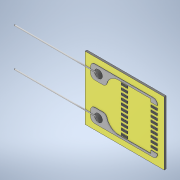
# Autodesk Inventor part: 應變規
Saved by Autodesk Inventor 2022 (Build 260153000, 153)
## iProperties
Created: 2023-03-14
Part Number: 應變規
Material: 一般
Document SubType Name: Modeling
Designer: User
Mass: 0.168829 g
Surface Area: 7.27926 cm^2
Volume: 0.168829 cm^3
Density: 1 g/cm^3
Appearance: 預設
Author: User
Autodesk Inventor part; units mm, degrees
ref_plane "XZ Plane" through (0, 0, 0) normal (0, 1, 0) x (-1, 0, 0)
ref_plane "XY Plane" through (0, 0, 0) normal (0, 0, 1) x (1, 0, 0)
sketch "草圖1" plane through (0, 0, 0) normal (0, 0, 1) x (1, 0, 0)
  line L0 (-10, 8) -> (10, 8)
  line L1 (10, 8) -> (10, -8)
  line L2 (10, -8) -> (-10, -8)
  line L3 (-10, -8) -> (-10, 8)
  line L4 (-14, 0) -> (14, 0) construction
  line L5 (0, -11.2) -> (0, 11.2) construction
  point P0 (0, 0)
  point P1 (0, 8)
  point P2 (10, 0)
  dimension "d0" = 16
  dimension "d1" = 20
  constraints: 8 end point, 2 midpoint, 2 parallel, 2 point on line, 1 horizontal, 1 perpendicular
  measures "d0" distance of L0.end L1.end
  measures "d1" distance of L0.start L0.end
extrude "擠出1" add sketch "草圖1" along normal blind 0.5
sketch "草圖2" plane through (0, 0, 0.5) normal (0, 0, 1) x (1, 0, 0)
  line L0 (-8, 6) -> (8, 6)
  line L1 (8, -6) -> (-8, -6)
  line L2 (-8, 6) -> (-4.5, 6)
  line L3 (-4.5, 6) -> (-4.5, 3)
  line L4 (-4.5, 3) -> (-8, 3)
  line L5 (-8, 3) -> (-8, 6)
  line L6 (-8, -6) -> (-4.5, -6)
  line L7 (-4.5, -6) -> (-4.5, -3)
  line L8 (-4.5, -3) -> (-8, -3)
  line L9 (-8, -3) -> (-8, -6)
  arc A0 (-1.5, 6) -> (-4.5, 3) centre (-1.5, 3) ccw
  arc A1 (-4.5, -3) -> (-1.5, -6) centre (-1.5, -3) ccw
  line L10 (-14, 0) -> (14, 0) construction
  line L11 (0, -11.2) -> (0, 11.2) construction
  line L12 (-8.5, 6.5) -> (8.3, 6.5)
  line L13 (8.3, -6.5) -> (-8.5, -6.5)
  line L14 (-8, 3) -> (-8.5, 3)
  line L15 (-8, -3) -> (-8.5, -3)
  line L16 (-8, -6) -> (-8, -3)
  line L17 (-8, 3) -> (-8, 6)
  line L18 (-8.5, 6.5) -> (-8.5, 3)
  line L19 (-8.5, -3) -> (-8.5, -6.5)
  line L20 (8.3, 6.5) -> (6.7, 6.5)
  line L21 (6.7, 6.5) -> (6.7, 5.5)
  line L22 (6.7, 5.5) -> (8.3, 5.5)
  line L23 (8.3, 5.5) -> (8.3, 6.5)
  line L24 (8.3, -6.5) -> (6.7, -6.5)
  line L25 (6.7, -6.5) -> (6.7, -5.5)
  line L26 (6.7, -5.5) -> (8.3, -5.5)
  line L27 (8.3, -5.5) -> (8.3, -6.5)
  line L28 (8.3, 6.5) -> (8.3, 5.5)
  line L29 (8.3, -5.5) -> (8.3, -6.5)
  line L30 (8.3, 6) -> (8.3, 5.5)
  line L31 (8.3, -5.5) -> (8.3, -6)
  line L32 (8, 6) -> (8, 5.5)
  line L33 (8, -5.5) -> (8, -6)
  line L34 (8, -6) -> (8, -5.5)
  line L35 (8, 5.5) -> (8, 6)
  point P0 (0, 0)
  point P1 (0, 6)
  point P2 (6.7, 6)
  point P3 (6.7, -6)
  dimension "d5" = 12
  dimension "d6" = 3
  dimension "d7" = 3
  dimension "d8" = 3.5
  dimension "d9" = 0.5
  dimension "d41" = 1
  dimension "d42" = 1
  dimension "d43" = 1.6
  dimension "d44" = 1.6
  constraints: 68 end point, 18 parallel, 12 perpendicular, 6 point on line, 5 horizontal, 4 point on circle, 4 tangent, 2 centre point, 2 midpoint, 2 vertical
  measures "d5" distance between parallel lines of L1 L0
  measures "d6" distance between parallel lines of L0 L4
  measures "d7" distance between parallel lines of L6 L8
  measures "d8" distance between parallel lines of L5 L3
  measures "d9" distance between parallel lines of L12 L0
  measures "d41" distance between parallel lines of L20 L22
  measures "d42" distance between parallel lines of L13 L26
  measures "d43" distance of L26.end L25.end
  measures "d44" distance of L21.end L22.end
extrude "擠出2" add sketch "草圖2" along normal blind 0.1
fillet "圓角1" radius 1 6 edges at (-4.5, 3, 0.55) (-4.5, -3, 0.55) (-8.5, -3, 0.55) (-8.5, 3, 0.55) (-8.5, 6.5, 0.55) (-8.5, -6.5, 0.55)
fillet "圓角2" radius 1 2 edges at (8.3, 6.5, 0.55) (8.3, -6.5, 0.55)
sketch "草圖3" plane through (0, 0, 0.5) normal (0, 0, 1) x (1, 0, 0)
  line L0 (0, -11.2) -> (0, 11.2) construction
  line L1 (-14, 0) -> (14, 0) construction
  line L2 (-0.8, 5.75) -> (0.8, 5.75)
  line L3 (0.8, 5.75) -> (0.8, 5.25)
  line L4 (0.8, 5.25) -> (-0.8, 5.25)
  line L5 (-0.8, 5.25) -> (-0.8, 5.75)
  line L6 (-0.8, 4.65) -> (0.8, 4.65)
  line L7 (0.8, 4.65) -> (0.8, 4.15)
  line L8 (0.8, 4.15) -> (-0.8, 4.15)
  line L9 (-0.8, 4.15) -> (-0.8, 4.65)
  line L10 (-0.8, 3.55) -> (0.8, 3.55)
  line L11 (0.8, 3.55) -> (0.8, 3.05)
  line L12 (0.8, 3.05) -> (-0.8, 3.05)
  line L13 (-0.8, 3.05) -> (-0.8, 3.55)
  line L14 (-0.8, 2.45) -> (0.8, 2.45)
  line L15 (0.8, 2.45) -> (0.8, 1.95)
  line L16 (0.8, 1.95) -> (-0.8, 1.95)
  line L17 (-0.8, 1.95) -> (-0.8, 2.45)
  line L18 (-0.8, 1.35) -> (0.8, 1.35)
  line L19 (0.8, 1.35) -> (0.8, 0.85)
  line L20 (0.8, 0.85) -> (-0.8, 0.85)
  line L21 (-0.8, 0.85) -> (-0.8, 1.35)
  line L22 (-0.8, 0.25) -> (0.8, 0.25)
  line L23 (0.8, 0.25) -> (0.8, -0.25)
  line L24 (0.8, -0.25) -> (-0.8, -0.25)
  line L25 (-0.8, -0.25) -> (-0.8, 0.25)
  line L26 (-0.8, -5.75) -> (0.8, -5.75)
  line L27 (0.8, -5.75) -> (0.8, -5.25)
  line L28 (0.8, -5.25) -> (-0.8, -5.25)
  line L29 (-0.8, -5.25) -> (-0.8, -5.75)
  line L30 (-0.8, -4.65) -> (0.8, -4.65)
  line L31 (0.8, -4.65) -> (0.8, -4.15)
  line L32 (0.8, -4.15) -> (-0.8, -4.15)
  line L33 (-0.8, -4.15) -> (-0.8, -4.65)
  line L34 (-0.8, -3.55) -> (0.8, -3.55)
  line L35 (0.8, -3.55) -> (0.8, -3.05)
  line L36 (0.8, -3.05) -> (-0.8, -3.05)
  line L37 (-0.8, -3.05) -> (-0.8, -3.55)
  line L38 (-0.8, -2.45) -> (0.8, -2.45)
  line L39 (0.8, -2.45) -> (0.8, -1.95)
  line L40 (0.8, -1.95) -> (-0.8, -1.95)
  line L41 (-0.8, -1.95) -> (-0.8, -2.45)
  line L42 (-0.8, -1.35) -> (0.8, -1.35)
  line L43 (0.8, -1.35) -> (0.8, -0.85)
  line L44 (0.8, -0.85) -> (-0.8, -0.85)
  line L45 (-0.8, -0.85) -> (-0.8, -1.35)
  point P0 (0, 0)
  point P1 (0, 0.85)
  point P2 (0, -0.25)
  point P3 (0.8, 0)
  point P4 (0, -0.85)
  dimension "d15" = 0.5
  dimension "d16" = 0.5
  dimension "d17" = 0.5
  dimension "d18" = 0.5
  dimension "d19" = 0.5
  dimension "d20" = 1.6
  dimension "d21" = 0.5
  dimension "d22" = 1.6
  dimension "d23" = 0.6
  dimension "d24" = 0.6
  dimension "d25" = 0.6
  dimension "d26" = 0.6
  dimension "d27" = 0.6
  constraints: 88 end point, 21 symmetric about line, 18 point on line, 12 parallel, 6 horizontal, 6 perpendicular, 3 midpoint
  measures "d15" distance between parallel lines of L4 L2
  measures "d16" distance of L6.end L7.end
  measures "d17" distance of L10.end L11.end
  measures "d18" distance of L14.end L15.end
  measures "d19" distance of L18.end L19.end
  measures "d20" distance of L18.start L18.end
  measures "d21" distance of L22.end L23.end
  measures "d22" distance of L22.start L22.end
  measures "d23" distance between parallel lines of L22 L20
  measures "d24" distance between parallel lines of L16 L18
  measures "d25" distance between parallel lines of L12 L14
  measures "d26" distance between parallel lines of L8 L10
  measures "d27" distance between parallel lines of L4 L6
extrude "擠出3" add sketch "草圖3" along normal blind 0.1
sketch "草圖5" plane through (0, 0, 0.5) normal (0, 0, 1) x (1, 0, 0)
  circle A0 centre (-6.5, 4.8) radius 1
  line L0 (0, -11.2) -> (0, 11.2) construction
  line L1 (-14, 0) -> (14, 0) construction
  circle A1 centre (-6.5, -4.8) radius 1
  point P0 (0, 0)
  dimension "d30" = 2
  dimension "d31" = 6.5
  dimension "d32" = 4.8
  constraints: 2 centre point, 1 symmetric about line, 1 other
  measures "d30" diameter of A0
  measures "d31" distance from line of L0 A0.centre
  measures "d32" distance from line of L1 A0.centre
extrude "擠出4" cut sketch "草圖5" along normal blind 1.65
ref_plane "工作平面1" through (-6.5, 0, 0) normal (1, 0, 0) x (0, 1, 0)
sketch "草圖6" plane through (-6.5, 0, 0) normal (1, 0, 0) x (0, 1, 0)
  line L0 (3.8, 0.6) -> (5.8, 0.6) projected
  line L1 (5.8, 0.5) -> (3.8, 0.5) projected
  arc A0 (4.8, 0.7383) -> (3.8, 0.5) centre (5.2194, -3.2397) ccw
  line L2 (4.8, 0.7383) -> (4.8, 0.5)
  line L3 (3.8, 0.5) -> (4.8, 0.5)
  constraints: 4 end point, 2 point on circle, 1 centre point, 1 collinear, 1 midpoint, 1 perpendicular
revolve "迴轉1" add sketch "草圖6" angle 360 about axis through (-6.5, 4.8, 0.7383) along (0, 0, -1)
mirror "鏡射1" about plane through (0, 0, 0) normal (0, 1, 0) of "迴轉1"
sketch "草圖7" plane through (-6.5, 0, 0) normal (1, 0, 0) x (0, 1, 0)
  circle A0 centre (4.8095, 0.5129) radius 0.15
  dimension "d38" = 0.3
  constraints: 1 centre point
  measures "d38" diameter of A0
extrude "擠出5" add sketch "草圖7" against normal blind 21.25
mirror "鏡射2" about plane through (0, 0, 0) normal (0, 1, 0) of "擠出5"
pattern_linear "矩形陣列1" count 2 spacing 7.5 along (1, 0, 0) of "擠出3"
